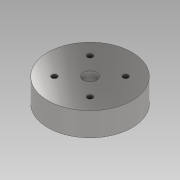
# Autodesk Inventor part: Stator
Saved by Autodesk Inventor 2020 (Build 240168000, 168)
## iProperties
Created: 2019-08-30
Part Number: Stator
Material: ステンレス鋼
Document SubType Name: Modeling
Designer: Ryohei
Density: 8 g/cm^3
Appearance: 半つや出し
Mass: 212.875 g
Surface Area: 65.8664 cm^2
Volume: 26.6094 cm^3
Author: Ryohei
Autodesk Inventor part; units mm, degrees
ref_plane "YZ Plane" through (0, 0, 0) normal (1, 0, 0) x (0, 1, 0)
ref_plane "XZ Plane" through (0, 0, 0) normal (0, 1, 0) x (-1, 0, 0)
ref_plane "XY Plane" through (0, 0, 0) normal (0, 0, 1) x (1, 0, 0)
sketch "スケッチ5" plane through (0, 0, 0) normal (0, 1, 0) x (-1, 0, 0)
  circle A0 centre (0, 0) radius 25
  dimension "d23" = 50
  constraints: 1 centre point, 1 coincident
  measures "d23" diameter of A0
extrude "押し出し2" add sketch "スケッチ5" along normal blind 14
sketch "スケッチ6" plane through (0, 14, 0) normal (0, 1, 0) x (1, 0, 0)
  circle A0 centre (0, 0) radius 4
  dimension "d26" = 8
  constraints: 1 centre point, 1 coincident
  measures "d26" diameter of A0
extrude "押し出し3" cut sketch "スケッチ6" against normal blind 14
sketch "スケッチ7" plane through (0, 14, 0) normal (0, 1, 0) x (1, 0, 0)
  line L0 (0, 0) -> (10.6066, 10.6066)
  line L1 (0, 0) -> (15, 0) construction
  point P0 (-10.6066, 10.6066)
  point P1 (-10.6066, -10.6066)
  point P2 (10.6066, -10.6066)
  dimension "d29" = 15
  dimension "d30" = 45
  dimension "d33" = 360
  constraints: 4 end point, 1 coincident, 1 equal length, 1 horizontal, 5 other
  measures "d29" distance of L0.start L0.end
  measures "d30" angle of L1 L0
hole "穴2" at (10.6066, 14, -10.6066) at (-10.6066, 14, -10.6066) at (-10.6066, 14, 10.6066) at (10.6066, 14, 10.6066) direction (0, -1, 0) diameter 3.242 depth 5 tip angle 118 thread size "M4x0.7" class "6H" standard "ISO Metric profile"
